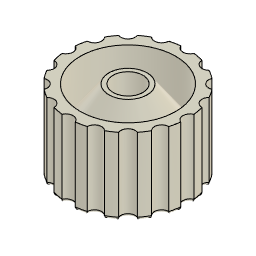
Display Knob (Autodesk Fusion 360 design; units mm, degrees)
Autodesk Fusion 360 part; units mm, degrees
note: some values were not read from the file. Set by a fixed rule: which sketch regions a step uses.
ref_plane "WorkPlane1" through (0, 0, 15) normal (0, 0, 1) x (1, 0, 0)
sketch "Sketch1" plane through (0, 0, 0) normal (0, 0, 1) x (1, 0, 0)
  circle A0 centre (0, 0) radius 12.5
  circle A1 centre (0, 0) radius 3.125
  circle A2 centre (0, 0) radius 10.5
  line L0 (0, 0) -> (0, -12.5) construction
  line L1 (0, -12.5) -> (0, -11.5) construction
  line L2 (0, -12.5) -> (0, -13) construction
  arc A3 (1.3846, -12.4231) -> (-1.3846, -12.4231) centre (0, -13) ccw
  arc A4 (6.0333, -10.9476) -> (3.4749, -12.0073) centre (4.9749, -12.0104) ccw
  arc A5 (9.7635, -7.8054) -> (7.8054, -9.7635) centre (9.1924, -9.1924) ccw
  arc A6 (12.0073, -3.4749) -> (10.9476, -6.0333) centre (12.0104, -4.9749) ccw
  arc A7 (12.4231, 1.3846) -> (12.4231, -1.3846) centre (13, 0) ccw
  arc A8 (10.9476, 6.0333) -> (12.0073, 3.4749) centre (12.0104, 4.9749) ccw
  arc A9 (7.8054, 9.7635) -> (9.7635, 7.8054) centre (9.1924, 9.1924) ccw
  arc A10 (3.4749, 12.0073) -> (6.0333, 10.9476) centre (4.9749, 12.0104) ccw
  arc A11 (-1.3846, 12.4231) -> (1.3846, 12.4231) centre (0, 13) ccw
  arc A12 (-6.0333, 10.9476) -> (-3.4749, 12.0073) centre (-4.9749, 12.0104) ccw
  arc A13 (-9.7635, 7.8054) -> (-7.8054, 9.7635) centre (-9.1924, 9.1924) ccw
  arc A14 (-12.0073, 3.4749) -> (-10.9476, 6.0333) centre (-12.0104, 4.9749) ccw
  arc A15 (-12.4231, -1.3846) -> (-12.4231, 1.3846) centre (-13, 0) ccw
  arc A16 (-10.9476, -6.0333) -> (-12.0073, -3.4749) centre (-12.0104, -4.9749) ccw
  arc A17 (-7.8054, -9.7635) -> (-9.7635, -7.8054) centre (-9.1924, -9.1924) ccw
  arc A18 (-3.4749, -12.0073) -> (-6.0333, -10.9476) centre (-4.9749, -12.0104) ccw
  dimension "d2" = 25
  dimension "d3" = 6.25
  dimension "d5" = 21
  dimension "d9" = 1.5
  dimension "d11" = 360
  constraint coincident A0.centre A1.centre
  constraint concentric A0 A1
  constraint coincident A0 L0.end
  constraint vertical L0
  constraint coincident L0 L1.end
  constraint parallel L0 L2
  constraint coincident A0 A3.end
  constraint coincident L2.end A3.centre
  constraint coincident A0 A3.start
  measures "d2" diameter of A0
  measures "d3" diameter of A1
  measures "d5" diameter of A2
  measures "d9" radius of A3
sketch "Sketch2" plane through (0, 0, 0) normal (0, 1, 0) x (1, 0, 0)
  line L0 (0, 0) -> (3.2994, 0)
  line L1 (3.2994, 0) -> (9, 0)
  arc A0 (3.2994, 0) -> (9, 0) centre (6.1497, 1) ccw
  line L2 (9, 0) -> (7.9672, -1.4127)
  line L3 (4.3322, -1.4127) -> (3.2994, 0)
  line L4 (6.1497, 0) -> (6.1497, -2.5) construction
  line L5 (6.1497, -2.5) -> (4.3322, -1.4127)
  line L6 (6.1497, -2.5) -> (7.9672, -1.4127)
  dimension "d26" = 1
  dimension "d27" = 1.75
  dimension "d30" = 1.75
  constraint coincident L0.start origin
  constraint horizontal L0
  constraint parallel L0 L1
  constraint coincident A0 L2.end
  constraint coincident A0 L3.start
  constraint midpoint L1 L4.start
  constraint perpendicular L1 L4
  measures "d26" distance of L1 A0.centre
  measures "d27" distance of L1.end L2.end
  measures "d30" distance of L0.end L3.start
extrude "Extrude1" add sketch "Sketch1" along normal blind 6 contours A0 A3 A4 A5 A6 A7 A8 A9 A10 A11 A12 A13 A14 A15 A16 A17 A18 | A1 | A2
revolve "Revolve1" cut sketch "Sketch2" angle 360 about axis through (0, 0, 1.75) along (0, 0, 1) contours L1 A0 L2 L3 L5 L6 | A0 L5 L6
fillet "Fillet1" radius 0.6 1 faces at (9.0501, 6.0808, 0)
sketch "Sketch3" plane through (0, 0, 6) normal (0, 0, 1) x (-1, 0, 0)
  arc A0 (-1.3846, 12.4231) -> (-3.4749, 12.0073) centre (0, 0) ccw
  arc A1 (-6.0333, 10.9476) -> (-3.4749, 12.0073) centre (-4.9749, 12.0104) ccw
  arc A2 (-6.0333, 10.9476) -> (-7.8054, 9.7635) centre (0, 0) ccw
  arc A3 (-9.7635, 7.8054) -> (-7.8054, 9.7635) centre (-9.1924, 9.1924) ccw
  arc A4 (-9.7635, 7.8054) -> (-10.9476, 6.0333) centre (0, 0) ccw
  arc A5 (-12.0073, 3.4749) -> (-10.9476, 6.0333) centre (-12.0104, 4.9749) ccw
  arc A6 (-12.0073, 3.4749) -> (-12.4231, 1.3846) centre (0, 0) ccw
  arc A7 (-12.4231, -1.3846) -> (-12.4231, 1.3846) centre (-13, 0) ccw
  arc A8 (-12.4231, -1.3846) -> (-12.0073, -3.4749) centre (0, 0) ccw
  arc A9 (-10.9476, -6.0333) -> (-12.0073, -3.4749) centre (-12.0104, -4.9749) ccw
  arc A10 (-10.9476, -6.0333) -> (-9.7635, -7.8054) centre (0, 0) ccw
  arc A11 (-7.8054, -9.7635) -> (-9.7635, -7.8054) centre (-9.1924, -9.1924) ccw
  arc A12 (-7.8054, -9.7635) -> (-6.0333, -10.9476) centre (0, 0) ccw
  arc A13 (-3.4749, -12.0073) -> (-6.0333, -10.9476) centre (-4.9749, -12.0104) ccw
  arc A14 (-3.4749, -12.0073) -> (-1.3846, -12.4231) centre (0, 0) ccw
  arc A15 (1.3846, -12.4231) -> (-1.3846, -12.4231) centre (0, -13) ccw
  arc A16 (1.3846, -12.4231) -> (3.4749, -12.0073) centre (0, 0) ccw
  arc A17 (6.0333, -10.9476) -> (3.4749, -12.0073) centre (4.9749, -12.0104) ccw
  arc A18 (6.0333, -10.9476) -> (7.8054, -9.7635) centre (0, 0) ccw
  arc A19 (9.7635, -7.8054) -> (7.8054, -9.7635) centre (9.1924, -9.1924) ccw
  arc A20 (9.7635, -7.8054) -> (10.9476, -6.0333) centre (0, 0) ccw
  arc A21 (12.0073, -3.4749) -> (10.9476, -6.0333) centre (12.0104, -4.9749) ccw
  arc A22 (12.0073, -3.4749) -> (12.4231, -1.3846) centre (0, 0) ccw
  arc A23 (12.4231, 1.3846) -> (12.4231, -1.3846) centre (13, 0) ccw
  arc A24 (12.4231, 1.3846) -> (12.0073, 3.4749) centre (0, 0) ccw
  arc A25 (10.9476, 6.0333) -> (12.0073, 3.4749) centre (12.0104, 4.9749) ccw
  arc A26 (10.9476, 6.0333) -> (9.7635, 7.8054) centre (0, 0) ccw
  arc A27 (7.8054, 9.7635) -> (9.7635, 7.8054) centre (9.1924, 9.1924) ccw
  arc A28 (7.8054, 9.7635) -> (6.0333, 10.9476) centre (0, 0) ccw
  arc A29 (3.4749, 12.0073) -> (6.0333, 10.9476) centre (4.9749, 12.0104) ccw
  arc A30 (3.4749, 12.0073) -> (1.3846, 12.4231) centre (0, 0) ccw
  arc A31 (-1.3846, 12.4231) -> (1.3846, 12.4231) centre (0, 13) ccw
  circle A32 centre (0, 0) radius 4
  circle A33 centre (0, 0) radius 10
  circle A34 centre (0, 0) radius 3.125
  dimension "d16" = 8
  dimension "d17" = 6.25
  constraint coincident A0.centre A2.centre
  constraint concentric A33 A34
  measures "d16" diameter of A32
  measures "d17" diameter of A34
extrude "Extrude2" add sketch "Sketch3" along normal blind 10 contours A32 | A33
chamfer "Chamfer1" distance 6 angle 55 1 edges at (9.3233, 3.6162, 16) measured on face at (-7.6595, 0.6521, 16)
extrude "Extrude3" add 1 faces at (6.1575, -8.8901, 6) along direction (0, 0, 1) blind 10
fillet "Fillet3" radius 1 1 edges at (-3.0761, 1.1931, 0)
